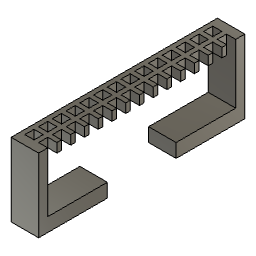
guard for a trailer part without grid v2 (Autodesk Fusion 360 design; units mm, degrees)
Autodesk Fusion 360 part; units mm, degrees
sketch "Sketch1" plane through (0, 0, 0) normal (0, 0, 1) x (1, 0, 0)
  line L0 (0, 0) -> (6, 0)
  line L1 (6, 0) -> (6, 2)
  line L2 (6, 2) -> (0, 2)
  line L3 (0, 2) -> (0, 0)
  line L4 (0, 2) -> (6, 2)
  line L5 (6, 2) -> (6, 15)
  line L6 (6, 15) -> (0, 15)
  line L7 (0, 15) -> (0, 2)
  line L8 (0, 15) -> (6, 15)
  line L9 (6, 15) -> (6, 30)
  line L10 (6, 30) -> (0, 30)
  line L11 (0, 30) -> (0, 15)
  line L12 (0, 30) -> (6, 30)
  line L13 (6, 30) -> (6, 43)
  line L14 (6, 43) -> (0, 43)
  line L15 (0, 43) -> (0, 30)
  line L16 (0, 43) -> (6, 43)
  line L17 (6, 43) -> (6, 45)
  line L18 (6, 45) -> (0, 45)
  line L19 (0, 45) -> (0, 43)
  dimension "d1" = 6
  dimension "d2" = 2
  dimension "d4" = 13
  dimension "d6" = 15
  dimension "d8" = 13
  dimension "d10" = 2
  constraint horizontal L0
  constraint vertical L1
  constraint horizontal L2
  constraint vertical L3
  constraint coincident L0.start L3.end
  constraint horizontal L4
  constraint vertical L5
  constraint horizontal L6
  constraint vertical L7
  constraint horizontal L8
  constraint vertical L9
  constraint horizontal L10
  constraint vertical L11
  constraint horizontal L12
  constraint vertical L13
  constraint horizontal L14
  constraint vertical L15
  constraint horizontal L16
  constraint vertical L17
  constraint horizontal L18
  constraint vertical L19
  measures "d1" distance of L0.start L0.end
  measures "d2" distance of L0.start L2.end
  measures "d4" distance of L2.end L6.end
  measures "d6" distance of L6.end L10.end
  measures "d8" distance of L10.end L14.end
  measures "d10" distance of L14.end L18.end
extrude "Extrude8" add sketch "Sketch1" along normal blind 3 contours L2 L4 L5 L6 L7 L8 | L10 L12 L13 L14 L15 L16 makes body 1 at (4, 6.3333, 0) makes body 2 at (2, 38.6667, 0)
extrude "Extrude9" add sketch "Sketch1" along normal blind 16 contours L0 L1 L2 L3 L4 | L14 L16 L17 L18 L19 bodies 1 2
sketch "Sketch4" plane through (0, 0, 16) normal (0, 0, 1) x (-1, 0, 0)
  line L0 (0, -45) -> (0, -43)
  line L1 (0, -43) -> (-6, -43)
  line L2 (-6, -43) -> (-6, -45)
  line L3 (-6, -45) -> (0, -45)
  line L4 (0, -43) -> (-1, -43)
  line L5 (-1, -43) -> (-1, -2)
  line L6 (-1, -2) -> (0, -2)
  line L7 (0, -2) -> (0, -43)
  line L8 (-3, -43) -> (-4, -43)
  line L9 (-4, -43) -> (-4, -2)
  line L10 (-4, -2) -> (-3, -2)
  line L11 (-3, -2) -> (-3, -43)
  line L12 (-1, -41) -> (-3, -41)
  line L13 (-3, -41) -> (-3, -40)
  line L14 (-3, -40) -> (-1, -40)
  line L15 (-1, -40) -> (-1, -41)
  line L16 (-1, -38) -> (-3, -38)
  line L17 (-3, -38) -> (-3, -37)
  line L18 (-3, -37) -> (-1, -37)
  line L19 (-1, -37) -> (-1, -38)
  line L20 (-1, -35) -> (-3, -35)
  line L21 (-3, -35) -> (-3, -34)
  line L22 (-3, -34) -> (-1, -34)
  line L23 (-1, -34) -> (-1, -35)
  line L24 (-1, -32) -> (-3, -32)
  line L25 (-3, -32) -> (-3, -31)
  line L26 (-3, -31) -> (-1, -31)
  line L27 (-1, -31) -> (-1, -32)
  line L28 (-1, -29) -> (-3, -29)
  line L29 (-3, -29) -> (-3, -28)
  line L30 (-3, -28) -> (-1, -28)
  line L31 (-1, -28) -> (-1, -29)
  line L32 (-1, -26) -> (-3, -26)
  line L33 (-3, -26) -> (-3, -25)
  line L34 (-3, -25) -> (-1, -25)
  line L35 (-1, -25) -> (-1, -26)
  line L36 (-1, -23) -> (-3, -23)
  line L37 (-3, -23) -> (-3, -22)
  line L38 (-3, -22) -> (-1, -22)
  line L39 (-1, -22) -> (-1, -23)
  line L40 (-1, -20) -> (-3, -20)
  line L41 (-3, -20) -> (-3, -19)
  line L42 (-3, -19) -> (-1, -19)
  line L43 (-1, -19) -> (-1, -20)
  line L44 (-1, -17) -> (-3, -17)
  line L45 (-3, -17) -> (-3, -16)
  line L46 (-3, -16) -> (-1, -16)
  line L47 (-1, -16) -> (-1, -17)
  line L48 (-1, -14) -> (-3, -14)
  line L49 (-3, -14) -> (-3, -13)
  line L50 (-3, -13) -> (-1, -13)
  line L51 (-1, -13) -> (-1, -14)
  line L52 (-1, -11) -> (-3, -11)
  line L53 (-3, -11) -> (-3, -10)
  line L54 (-3, -10) -> (-1, -10)
  line L55 (-1, -10) -> (-1, -11)
  line L56 (-1, -8) -> (-3, -8)
  line L57 (-3, -8) -> (-3, -7)
  line L58 (-3, -7) -> (-1, -7)
  line L59 (-1, -7) -> (-1, -8)
  line L60 (-1, -5) -> (-3, -5)
  line L61 (-3, -5) -> (-3, -4)
  line L62 (-3, -4) -> (-1, -4)
  line L63 (-1, -4) -> (-1, -5)
  line L64 (-4, -23) -> (-6, -23)
  line L65 (-6, -23) -> (-6, -22)
  line L66 (-6, -22) -> (-4, -22)
  line L67 (-4, -22) -> (-4, -23)
  line L68 (-4, -20) -> (-6, -20)
  line L69 (-6, -20) -> (-6, -19)
  line L70 (-6, -19) -> (-4, -19)
  line L71 (-4, -19) -> (-4, -20)
  line L72 (-4, -17) -> (-6, -17)
  line L73 (-6, -17) -> (-6, -16)
  line L74 (-6, -16) -> (-4, -16)
  line L75 (-4, -16) -> (-4, -17)
  line L76 (-4, -14) -> (-6, -14)
  line L77 (-6, -14) -> (-6, -13)
  line L78 (-6, -13) -> (-4, -13)
  line L79 (-4, -13) -> (-4, -14)
  line L80 (-4, -11) -> (-6, -11)
  line L81 (-6, -11) -> (-6, -10)
  line L82 (-6, -10) -> (-4, -10)
  line L83 (-4, -10) -> (-4, -11)
  line L84 (-4, -8) -> (-6, -8)
  line L85 (-6, -8) -> (-6, -7)
  line L86 (-6, -7) -> (-4, -7)
  line L87 (-4, -7) -> (-4, -8)
  line L88 (-4, -5) -> (-6, -5)
  line L89 (-6, -5) -> (-6, -4)
  line L90 (-6, -4) -> (-4, -4)
  line L91 (-4, -4) -> (-4, -5)
  line L92 (-4, -26) -> (-6, -26)
  line L93 (-6, -26) -> (-6, -25)
  line L94 (-6, -25) -> (-4, -25)
  line L95 (-4, -25) -> (-4, -26)
  line L96 (-4, -29) -> (-6, -29)
  line L97 (-6, -29) -> (-6, -28)
  line L98 (-6, -28) -> (-4, -28)
  line L99 (-4, -28) -> (-4, -29)
  line L100 (-4, -32) -> (-6, -32)
  line L101 (-6, -32) -> (-6, -31)
  line L102 (-6, -31) -> (-4, -31)
  line L103 (-4, -31) -> (-4, -32)
  line L104 (-4, -35) -> (-6, -35)
  line L105 (-6, -35) -> (-6, -34)
  line L106 (-6, -34) -> (-4, -34)
  line L107 (-4, -34) -> (-4, -35)
  line L108 (-4, -38) -> (-6, -38)
  line L109 (-6, -38) -> (-6, -37)
  line L110 (-6, -37) -> (-4, -37)
  line L111 (-4, -37) -> (-4, -38)
  line L112 (-4, -41) -> (-6, -41)
  line L113 (-6, -41) -> (-6, -40)
  line L114 (-6, -40) -> (-4, -40)
  line L115 (-4, -40) -> (-4, -41)
  dimension "d44" = 41
  dimension "d45" = 1
  dimension "d46" = 41
  constraint horizontal L4
  constraint vertical L5
  constraint horizontal L6
  constraint vertical L7
  constraint coincident L0.end L1.start
  constraint horizontal L8
  constraint vertical L9
  constraint horizontal L10
  constraint vertical L11
  constraint midpoint L1 L8.start
  constraint horizontal L12
  constraint vertical L13
  constraint horizontal L14
  constraint vertical L15
  constraint coincident L11 L13.end
  constraint coincident L5 L12.start
  constraint horizontal L16
  constraint vertical L17
  constraint horizontal L18
  constraint vertical L19
  constraint coincident L11 L17.end
  constraint coincident L5 L16.start
  constraint horizontal L20
  constraint vertical L21
  constraint horizontal L22
  constraint vertical L23
  constraint coincident L11 L21.end
  constraint coincident L5 L20.start
  constraint horizontal L24
  constraint vertical L25
  constraint horizontal L26
  constraint vertical L27
  constraint coincident L11 L25.end
  constraint coincident L5 L24.start
  constraint horizontal L28
  constraint vertical L29
  constraint horizontal L30
  constraint vertical L31
  constraint coincident L11 L29.end
  constraint coincident L5 L28.start
  constraint horizontal L32
  constraint vertical L33
  constraint horizontal L34
  constraint vertical L35
  constraint coincident L11 L33.end
  constraint coincident L5 L32.start
  constraint horizontal L36
  constraint vertical L37
  constraint horizontal L38
  constraint vertical L39
  constraint coincident L11 L37.end
  constraint coincident L5 L36.start
  constraint horizontal L40
  constraint vertical L41
  constraint horizontal L42
  constraint vertical L43
  constraint coincident L11 L41.end
  constraint coincident L5 L40.start
  constraint horizontal L44
  constraint vertical L45
  constraint horizontal L46
  constraint vertical L47
  constraint coincident L11 L45.end
  constraint coincident L5 L44.start
  constraint horizontal L48
  constraint vertical L49
  constraint horizontal L50
  constraint vertical L51
  constraint coincident L11 L49.end
  constraint coincident L5 L48.start
  constraint horizontal L52
  constraint vertical L53
  constraint horizontal L54
  constraint vertical L55
  constraint coincident L11 L53.end
  constraint coincident L5 L52.start
  constraint horizontal L56
  constraint vertical L57
  constraint horizontal L58
  constraint vertical L59
  constraint coincident L11 L57.end
  constraint coincident L5 L56.start
  constraint horizontal L60
  constraint vertical L61
  constraint horizontal L62
  constraint vertical L63
  constraint coincident L11 L61.end
  constraint coincident L5 L60.start
  constraint horizontal L64
  constraint vertical L65
  constraint horizontal L66
  constraint vertical L67
  constraint coincident L9 L64.start
  constraint horizontal L68
  constraint vertical L69
  constraint horizontal L70
  constraint vertical L71
  constraint coincident L9 L68.start
  constraint horizontal L72
  constraint vertical L73
  constraint horizontal L74
  constraint vertical L75
  constraint coincident L9 L72.start
  constraint horizontal L76
  constraint vertical L77
  constraint horizontal L78
  constraint vertical L79
  constraint coincident L9 L76.start
  constraint horizontal L80
  constraint vertical L81
  constraint horizontal L82
  constraint vertical L83
  constraint coincident L9 L80.start
  constraint horizontal L84
  constraint vertical L85
  constraint horizontal L86
  constraint vertical L87
  constraint coincident L9 L84.start
  constraint horizontal L88
  constraint vertical L89
  constraint horizontal L90
  constraint vertical L91
  constraint coincident L9 L88.start
  constraint horizontal L92
  constraint vertical L93
  constraint horizontal L94
  constraint vertical L95
  constraint coincident L9 L92.start
  constraint horizontal L96
  constraint vertical L97
  constraint horizontal L98
  constraint vertical L99
  constraint coincident L9 L96.start
  constraint horizontal L100
  constraint vertical L101
  constraint horizontal L102
  constraint vertical L103
  constraint coincident L9 L100.start
  constraint horizontal L104
  constraint vertical L105
  constraint horizontal L106
  constraint vertical L107
  constraint coincident L9 L104.start
  constraint horizontal L108
  constraint vertical L109
  constraint horizontal L110
  constraint vertical L111
  constraint coincident L9 L108.start
  constraint horizontal L112
  constraint vertical L113
  constraint horizontal L114
  constraint vertical L115
  constraint coincident L9 L112.start
  measures "d44" distance of L0.end L6.end
  measures "d45" distance of L8.start L8.end
  measures "d46" distance of L8.start L10.end
extrude "Extrude10" add sketch "Sketch4" against normal blind 2 contours L1 L4 L5 L6 L7 L15 L19 L23 L27 L31 L35 L39 L43 L47 L51 L55 L59 L63 | L1 L8 L9 L10 L11 L13 L17 L21 L25 L29 L33 L37 L41 L45 L49 L53 L57 L61 L67 L71 L75 L79 L83 L87 L91 L95 L99 L103 L107 L111 L115 | L5 L11 L12 L13 L14 L15 | L5 L11 L60 L61 L62 L63 | L5 L11 L16 L17 L18 L19 | L5 L11 L56 L57 L58 L59 | L5 L11 L20 L21 L22 L23 | L5 L11 L52 L53 L54 L55 | L5 L11 L24 L25 L26 L27 | L5 L11 L48 L49 L50 L51 | L5 L11 L28 L29 L30 L31 | L5 L11 L44 L45 L46 L47 | L5 L11 L32 L33 L34 L35 | L5 L11 L40 L41 L42 L43 | L5 L11 L36 L37 L38 L39 bodies 1 2
extrude "Extrude11" add sketch "Sketch4" against normal blind 2 contours L9 L112 L113 L114 L115 | L9 L108 L109 L110 L111 | L9 L88 L89 L90 L91 | L9 L104 L105 L106 L107 | L9 L84 L85 L86 L87 | L9 L100 L101 L102 L103 | L9 L80 L81 L82 L83 | L9 L96 L97 L98 L99 | L9 L76 L77 L78 L79 | L9 L92 L93 L94 L95 | L9 L72 L73 L74 L75 | L9 L64 L65 L66 L67 | L9 L68 L69 L70 L71 bodies 1
